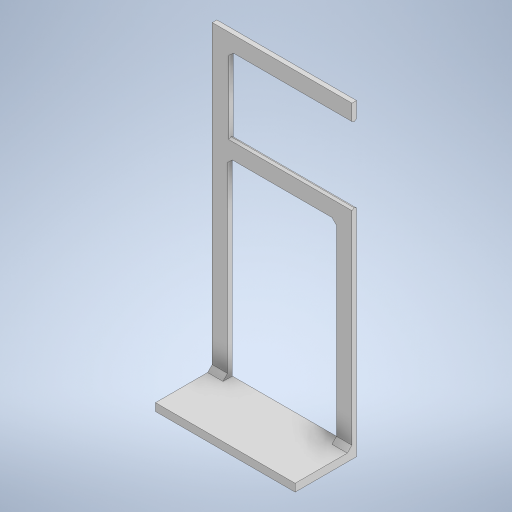
# Autodesk Inventor part: PiScanMiniDomeHolder
Saved by Autodesk Inventor 2023.2 (Build 272271000, 271)
## iProperties
Created: 2023-04-25
Part Number: PiScanMiniDomeHolder
Material: Generisch
Document SubType Name: Modeling
Designer: hangel
Density: 1 g/cm^3
Appearance: Vorgabe
Author: hangel
Autodesk Inventor part; units mm, degrees
ref_plane "YZ Plane" through (0, 0, 0) normal (1, 0, 0) x (0, 1, 0)
ref_plane "XZ Plane" through (0, 0, 0) normal (0, 1, 0) x (-1, 0, 0)
ref_plane "XY Plane" through (0, 0, 0) normal (0, 0, 1) x (1, 0, 0)
sketch "Skizze1" plane through (0, 0, 0) normal (0, 0, 1) x (1, 0, 0)
  line L0 (-45.5, 35.5) -> (45.5, 35.5)
  line L1 (45.5, 35.5) -> (45.5, -35.5)
  line L2 (45.5, -35.5) -> (-45.5, -35.5)
  line L3 (-45.5, -35.5) -> (-45.5, 35.5)
  line L4 (-45.5, 35.5) -> (45.5, -35.5) construction
  line L5 (45.5, 35.5) -> (-45.5, -35.5) construction
  line L6 (-34.8, 25.15) -> (45.5, 25.15)
  line L7 (-34.8, -25.15) -> (45.5, -25.15)
  line L8 (0, 0) -> (46.8412, 0)
  line L9 (-34.8, 25.15) -> (-34.8, -25.15)
  line L10 (-31.8, 25.15) -> (-40.5715, 16.3785)
  line L11 (-31.8, 25.15) -> (-19.3953, 25.15) construction
  point P0 (-34.8, 22.15)
  dimension "d0" = 91
  dimension "d1" = 71
  dimension "d4" = 80.3
  dimension "d5" = 50.3
  dimension "d23" = 135
  dimension "d24" = 3
  constraints: 24 end point, 3 horizontal, 3 perpendicular, 3 point on line, 2 equal length, 2 midpoint, 2 parallel, 1 vertical, 1 other
  measures "d0" distance of L1.end L2.end
  measures "d1" distance of L0.end L1.end
  measures "d4" distance of L6.start L6.end
  measures "d5" diameter of L6 L8
  measures "d23" angle of L10 L11
  measures "d24" distance from line of L10.start L9
extrude "Extrusion1" add sketch "Skizze1" along normal mid plane 3 contours L0 L1 L6 L9 L7 L2 L3 | L10 L9 L6
sketch "Skizze3" plane through (45.5, 25.15, 1.5) normal (1, 0, 0) x (0, 0, -1)
  line L0 (3, 0) -> (0, 0) projected
  line L1 (0, 0) -> (1.5, -0.866)
  line L2 (0, 0) -> (1.5, 0) construction
  line L3 (3, -50.3) -> (0, -50.3) projected
  line L4 (1.5, 0) -> (1.5, -50.3)
  line L5 (1.5, -0.866) -> (3, 0)
  line L6 (1.5, -25.15) -> (8.6012, -25.15)
  line L7 (0, -50.3) -> (1.5, -49.434)
  line L8 (1.5, -49.434) -> (3, -50.3)
  dimension "d7" = 30
  constraints: 14 end point, 2 horizontal, 1 midpoint, 1 point on line, 1 symmetric about line, 1 vertical
  measures "d7" angle of L1 L0
extrude "Extrusion2" add sketch "Skizze3" against normal up to surface (80.3 mm away)
sketch "Skizze4" plane through (-45.5, -35.5, 1.5) normal (0, -1, 0) x (1, 0, 0)
  line L0 (0, 0) -> (91, 0) projected
  line L1 (91, -3) -> (0, -3) projected
  line L2 (0, 0) -> (10, 0)
  line L3 (10, 0) -> (10, -3)
  line L4 (10, -3) -> (0, -3)
  line L5 (0, -3) -> (0, 0)
  line L6 (91, -3) -> (91, 0) projected
  line L7 (91, -3) -> (81, -3)
  line L8 (81, -3) -> (81, 0)
  line L9 (81, 0) -> (91, 0)
  line L10 (91, 0) -> (91, -3)
  point P0 (45.5, -1.5)
  point P1 (81, 0)
  point P2 (81, -3)
  dimension "d10" = 10
  dimension "d11" = 10
  constraints: 16 end point, 4 parallel, 2 horizontal, 2 perpendicular, 2 point on line
  measures "d10" distance of L3.end L4.end
  measures "d11" distance of L8.end L9.end
extrude "Extrusion3" add sketch "Skizze4" along normal blind 130 contours L0 L3 L1 L5 | L0 L6 L1 L8
chamfer "Fase1" distance 3 angle 45 2 edges at (-35.5, -35.5, 0) (35.5, -35.5, 0)
sketch "Skizze6" plane through (0, 0, -1.5) normal (0, 0, -1) x (-1, 0, 0)
  line L0 (45.5, 35.5) -> (45.5, -165.5) projected
  line L1 (-45.5, -25.15) -> (-45.5, -165.5) projected
  line L2 (45.5, -165.5) -> (-45.5, -165.5)
  line L3 (-45.5, -165.5) -> (-45.5, -160.5)
  line L4 (-45.5, -160.5) -> (45.5, -160.5)
  line L5 (45.5, -160.5) -> (45.5, -165.5)
  point P0 (0, 0)
  dimension "d20" = 5
  constraints: 8 end point, 2 parallel, 1 horizontal, 1 perpendicular, 1 point on line
  measures "d20" distance of L2.end L3.end
extrude "Extrusion5" add sketch "Skizze6" against normal blind 40
chamfer "Fase2" distance 3 angle 45 2 edges at (-40.5, -160.5, 1.5) (40.5, -160.5, 1.5)
equation "\"d11\" = d10"
